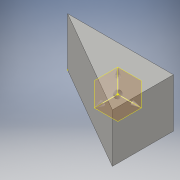
# Autodesk Inventor part: Wedge
Saved by Autodesk Inventor 2016 (Build 200138000, 138)
## iProperties
Created: 2015-09-10
Part Number: Wedge
Material: Generic
Document SubType Name: Modeling
Designer: Kanishka
Density: 1 g/cm^3
Appearance: Default
Mass: 10825.3 g
Surface Area: 3448.56 cm^2
Volume: 10825.3 cm^3
Author: Kanishka
Autodesk Inventor part; units mm, degrees
ref_plane "YZ Plane" through (0, 0, 0) normal (1, 0, 0) x (0, 1, 0)
ref_plane "XZ Plane" through (0, 0, 0) normal (0, 1, 0) x (-1, 0, 0)
ref_plane "XY Plane" through (0, 0, 0) normal (0, 0, 1) x (1, 0, 0)
sketch "Sketch2" plane through (0, 0, 0) normal (0, 1, 0) x (-1, 0, 0)
  line L0 (0, 0) -> (-433.0127, 250)
  line L1 (0, 0) -> (500, 0) construction
  line L2 (-433.0127, 250) -> (-433.0127, 0)
  line L3 (-433.0127, 0) -> (0, 0)
  dimension "d4" = 500
  dimension "d5" = 150
  constraints: 8 end point, 1 equal length, 1 horizontal, 1 perpendicular, 1 vertical
  measures "d4" distance of L0.start L0.end
  measures "d5" angle of L1 L0
extrude "Extrusion2" add sketch "Sketch2" along normal blind 200
sketch "Sketch3" plane through (0, 0, 0) normal (0, -1, 0) x (1, 0, 0)
  point P0 (0, 0)
body "Solid2"
